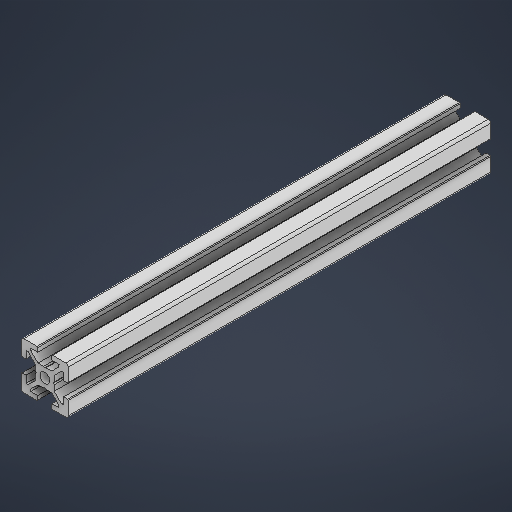
# Autodesk Inventor part: 20x20_180mm
Saved by Autodesk Inventor 2027 (Build 310192060, 192F)
## iProperties
Created: 2026-07-17
Part Number: 20x20_180mm
Material: Generic
Document SubType Name: Modeling
Designer: efloy
Density: 1 g/cm^3
Appearance: Default
Author: efloy
Autodesk Inventor part; units mm, degrees
ref_plane "YZ Plane" through (0, 0, 0) normal (1, 0, 0) x (0, 1, 0)
ref_plane "XZ Plane" through (0, 0, 0) normal (0, 1, 0) x (-1, 0, 0)
ref_plane "XY Plane" through (0, 0, 0) normal (0, 0, 1) x (1, 0, 0)
sketch "Sketch1" plane through (0, 0, 0) normal (0, 0, 1) x (1, 0, 0)
  line L0 (-13.429, -0.3286) -> (10.571, -0.3286)
  line L1 (-1.429, 11.6714) -> (-1.429, -12.3286)
  line L2 (5.6317, 5.6714) -> (2.571, 2.6107)
  line L3 (6.571, 5.6714) -> (6.571, 2.6714)
  line L4 (4.571, 6.7321) -> (1.5103, 3.6714)
  line L5 (-9.429, 5.6714) -> (-9.429, 2.6714)
  line L6 (-8.4897, 5.6714) -> (-5.429, 2.6107)
  line L7 (-7.429, 6.732) -> (-4.3683, 3.6714)
  line L8 (8.571, 8.6714) -> (8.571, 2.9714)
  line L9 (-11.429, 8.6714) -> (-11.429, 2.9714)
  line L10 (5.6317, -6.3286) -> (2.571, -3.2679)
  line L11 (1.871, -10.3286) -> (7.571, -10.3286)
  line L12 (-8.4897, -6.3286) -> (-5.429, -3.2679)
  line L13 (-7.429, -8.3286) -> (-4.429, -8.3286)
  line L14 (-7.429, -7.3893) -> (-4.3683, -4.3286)
  line L15 (-10.429, -10.3286) -> (-4.729, -10.3286)
  arc A0 (-11.129, -3.3286) -> (-11.429, -3.6286) centre (-11.129, -3.6286) ccw
  line L16 (-9.429, -6.3286) -> (-9.429, -3.3286)
  line L17 (-7.429, -7.3893) -> (-7.429, -8.3286)
  line L18 (-11.429, -3.6286) -> (-11.429, -9.3286)
  arc A1 (-11.429, -9.3286) -> (-10.429, -10.3286) centre (-10.429, -9.3286) ccw
  line L19 (-9.004, -10.3286) -> (-9.004, -10.3285)
  line L20 (-9.429, -6.3286) -> (-8.4897, -6.3286)
  line L21 (-11.129, -3.3286) -> (-9.429, -3.3286)
  line L22 (-11.129, 2.6714) -> (-9.429, 2.6714)
  arc A2 (-11.429, 2.9714) -> (-11.129, 2.6714) centre (-11.129, 2.9714) ccw
  arc A3 (-4.729, -10.3286) -> (-4.429, -10.0286) centre (-4.729, -10.0286) ccw
  line L23 (-4.429, -10.0286) -> (-4.429, -8.3286)
  line L24 (4.571, -7.3893) -> (4.571, -8.3286)
  line L25 (4.571, -8.3286) -> (1.571, -8.3286)
  arc A4 (1.571, -10.0286) -> (1.871, -10.3286) centre (1.871, -10.0286) ccw
  line L26 (1.571, -10.0286) -> (1.571, -8.3286)
  line L27 (4.571, -7.3893) -> (1.5103, -4.3286)
  circle A5 centre (-1.429, -0.3286) radius 2.1
  arc A6 (8.571, -3.6286) -> (8.271, -3.3286) centre (8.271, -3.6286) ccw
  line L28 (6.571, -6.3286) -> (6.571, -3.3286)
  line L29 (8.571, -3.6286) -> (8.571, -9.3286)
  arc A7 (7.571, -10.3286) -> (8.571, -9.3286) centre (7.571, -9.3286) ccw
  line L30 (5.6317, -6.3286) -> (6.571, -6.3286)
  line L31 (8.271, -3.3286) -> (6.571, -3.3286)
  line L32 (8.271, 2.6714) -> (6.571, 2.6714)
  arc A8 (8.271, 2.6714) -> (8.571, 2.9714) centre (8.271, 2.9714) ccw
  line L33 (1.871, 9.6714) -> (7.571, 9.6714)
  line L34 (-10.429, 9.6714) -> (-4.729, 9.6714)
  arc A9 (-4.429, 9.3714) -> (-4.729, 9.6714) centre (-4.729, 9.3714) ccw
  line L35 (-7.429, 7.6714) -> (-4.429, 7.6714)
  arc A10 (-10.429, 9.6714) -> (-11.429, 8.6714) centre (-10.429, 8.6714) ccw
  line L36 (-9.429, 5.6714) -> (-8.4897, 5.6714)
  line L37 (-7.429, 7.6714) -> (-7.429, 6.732)
  line L38 (-4.429, 9.3714) -> (-4.429, 7.6714)
  line L39 (1.571, 9.3714) -> (1.571, 7.6714)
  line L40 (4.571, 7.6714) -> (1.571, 7.6714)
  line L41 (4.571, 7.6714) -> (4.571, 6.7321)
  arc A11 (1.871, 9.6714) -> (1.571, 9.3714) centre (1.871, 9.3714) ccw
  arc A12 (8.571, 8.6714) -> (7.571, 9.6714) centre (7.571, 8.6714) ccw
  line L42 (5.6317, 5.6714) -> (6.571, 5.6714)
  line L43 (-5.429, 2.6107) -> (-5.429, 0.191)
  line L44 (2.571, 2.6107) -> (2.571, 0.191)
  line L45 (-4.3683, 3.6714) -> (-1.9486, 3.6714)
  line L46 (-4.3683, -4.3286) -> (-1.9486, -4.3286)
  line L47 (-1.429, 3.3714) -> (-1.9486, 3.6714)
  line L48 (-1.429, 3.3714) -> (-0.9094, 3.6714)
  line L49 (-0.9094, 3.6714) -> (1.5103, 3.6714)
  line L50 (-5.129, -0.3286) -> (-5.429, -0.8482)
  line L51 (-5.129, -0.3286) -> (-5.429, 0.191)
  line L52 (-1.429, -4.0286) -> (-0.9094, -4.3286)
  line L53 (-1.429, -4.0286) -> (-1.9486, -4.3286)
  line L54 (2.271, -0.3286) -> (2.571, 0.191)
  line L55 (2.271, -0.3286) -> (2.571, -0.8482)
  line L56 (2.571, -0.8482) -> (2.571, -3.2679)
  line L57 (-0.9094, -4.3286) -> (1.5103, -4.3286)
  line L58 (-5.429, -0.8482) -> (-5.429, -3.2679)
  point P0 (2.271, -0.3286)
  point P1 (5.6317, 5.6714)
  point P2 (8.271, 2.6714)
  point P3 (8.571, 2.9714)
  point P4 (1.871, 9.6714)
  point P5 (1.571, 9.3714)
  point P6 (-1.429, 3.3714)
  point P7 (-4.429, 9.3714)
  point P8 (-11.429, 2.9714)
  point P9 (-11.129, 2.6714)
  point P10 (-8.4897, 5.6714)
  point P11 (-5.129, -0.3286)
  point P12 (-8.4897, -6.3286)
  point P13 (-11.129, -3.3286)
  point P14 (-11.429, -3.6286)
  point P15 (-4.729, -10.3286)
  point P16 (-4.429, -10.0286)
  point P17 (-7.429, -7.3893)
  point P18 (-1.429, -4.0286)
  point P19 (4.571, -7.3893)
  point P20 (1.571, -10.0286)
  point P21 (1.871, -10.3286)
  point P22 (8.571, -3.6286)
  point P23 (8.271, -3.3286)
  point P24 (5.6317, -6.3286)
  dimension "d0" = 20
  dimension "d1" = 20
  constraints: 118 end point, 24 point on circle, 13 centre point
  measures "d0" distance between parallel lines of L15 L34
  measures "d1" distance between parallel lines of L18 L29
extrude "Extrusion1" add sketch "Sketch1" along normal blind 180 contours A5 L1 L48 L49 L4 L41 L40 L39 A11 L33 A12 L8 A8 L32 L3 L42 L2 L44 L54 L0 | L0 L55 L56 L10 L30 L28 L31 A6 L29 A7 L11 A4 L26 L25 L24 L27 L57 L52 L1 A5 | A5 L0 L51 L43 L6 L36 L5 L22 A2 L9 A10 L34 A9 L38 L35 L37 L7 L45 L47 L1 | L1 L53 L46 L14 L17 L13 L23 A3 L15 A1 L18 A0 L21 L16 L20 L12 L58 L50 L0 A5
body "Solid1"
